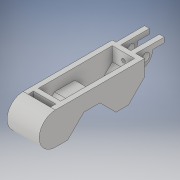
# Autodesk Inventor part: index
Saved by Autodesk Inventor 2019 (Build 230136000, 136)
## iProperties
Created: 2018-10-13
Part Number: index
Material: Generic
Document SubType Name: Modeling
Designer: jerem
Density: 1 g/cm^3
Appearance: Default
Author: jerem
Autodesk Inventor part; units mm, degrees
ref_plane "YZ Plane" through (0, 0, 0) normal (1, 0, 0) x (0, 1, 0)
ref_plane "XZ Plane" through (0, 0, 0) normal (0, 1, 0) x (-1, 0, 0)
sketch "Sketch2" plane through (0, 0, 0) normal (1, 0, 0) x (0, 1, 0)
  line L0 (0, 0) -> (0, -5)
  line L1 (13, 0) -> (13, -18)
  arc A0 (13, 0) -> (0, 0) centre (6.5, 0) ccw
  line L2 (-3.1385, 0) -> (18.8309, 0) projected
  line L3 (0, -54.8723) -> (0, 16.7287) projected
  line L4 (0, -5) -> (6.5, -11.5)
  line L5 (0, -5) -> (9.1924, -5) construction
  line L6 (6.5, -11.5) -> (6.5, -18)
  line L7 (6.5, -18) -> (0, -24.5)
  line L8 (6.5, -18) -> (15.6924, -18) construction
  line L9 (0, -24.5) -> (0, -29.5)
  line L10 (0, -29.5) -> (6.5, -36)
  line L11 (0, -29.5) -> (9.1924, -29.5) construction
  line L12 (13, -18) -> (13, -36)
  line L13 (13, -36) -> (13, -42.5)
  arc A1 (6.5, -36) -> (13, -42.5) centre (11.1419, -37.8581) ccw
  circle A2 centre (9.75, -40) radius 1.625
  dimension "d3" = 18
  dimension "d4" = 13
  dimension "d9" = 45
  dimension "d10" = 6.5
  dimension "d11" = 5
  dimension "d12" = 6.5
  dimension "d13" = 135
  dimension "d14" = 6.5
  dimension "d15" = 5
  dimension "d16" = 45
  dimension "d17" = 6.5
  dimension "d18" = 18
  dimension "d19" = 6.5
  dimension "d20" = 5
  dimension "d21" = 3.25
  dimension "d22" = 3.25
  dimension "d23" = 2.5
  constraints: 24 end point, 5 vertical, 4 point on circle, 3 centre point, 3 equal length, 3 horizontal, 2 point on line, 2 tangent, 1 collinear
  measures "d3" distance of L1.start L1.end
  measures "d4" distance between parallel lines of L1 L0
  measures "d9" angle of L4 L5
  measures "d10" horizontal distance of L4.end L0.end
  measures "d11" distance of L0.start L0.end
  measures "d12" distance of L4.end L6.end
  measures "d13" angle of L7 L8
  measures "d14" horizontal distance of L7.end L6.end
  measures "d15" distance of L7.end L9.end
  measures "d16" angle of L10 L11
  measures "d17" horizontal distance of L10.end L9.end
  measures "d18" distance of L1.end L12.end
  measures "d19" distance of L12.end L13.end
  measures "d20" radius of A1
  measures "d21" diameter of A2
  measures "d22" horizontal distance of A2.centre L13.end
  measures "d23" vertical distance of L13.end A2.centre
extrude "Extrusion1" add sketch "Sketch2" along normal mid plane 13 contours L2 L1 L12 L13 A1 L10 L3 L7 L6 L4 L0 | A0 L2
sketch "Sketch3" plane through (-6.5, 13, 0) normal (0, 1, 0) x (1, 0, 0)
  line L0 (0, 36) -> (13, 36) projected
  line L1 (0, 43) -> (1.5, 43)
  line L2 (1.5, 43) -> (1.5, 36)
  line L3 (1.5, 36) -> (0, 36)
  line L4 (0, 36) -> (0, 43)
  line L5 (0, 0) -> (0, 42.5) projected
  line L6 (3.5, 43) -> (7.5, 43)
  line L7 (7.5, 43) -> (7.5, 36)
  line L8 (7.5, 36) -> (3.5, 36)
  line L9 (3.5, 36) -> (3.5, 43)
  line L10 (9.5, 43) -> (13, 43)
  line L11 (13, 43) -> (13, 36)
  line L12 (13, 36) -> (9.5, 36)
  line L13 (9.5, 36) -> (9.5, 43)
  line L14 (13, 42.5) -> (13, 0) projected
  point P0 (6.5, 0)
  dimension "d47" = 1.5
  dimension "d48" = 7
  dimension "d49" = 4
  dimension "d50" = 7
  dimension "d51" = 2
  dimension "d52" = 7
  dimension "d53" = 2
  constraints: 24 end point, 6 parallel, 5 collinear, 3 horizontal, 3 perpendicular
  measures "d47" distance of L2.end L3.end
  measures "d48" distance of L1.end L2.end
  measures "d49" distance of L7.end L8.end
  measures "d50" distance of L6.end L7.end
  measures "d51" distance between parallel lines of L2 L9
  measures "d52" distance of L10.end L11.end
  measures "d53" distance between parallel lines of L13 L7
extrude "Extrusion2" cut sketch "Sketch3" against normal blind 13
ref_plane "Work Plane1" through (4.5, 0, 0) normal (1, 0, 0) x (0, 0, -1)
sketch "Sketch4" plane through (4.5, 0, 0) normal (1, 0, 0) x (0, 0, -1)
  arc A0 (0, 13) -> (0, 0) centre (0, 6.5) ccw projected
  line L0 (0, 13) -> (36, 13) projected
  line L1 (36, 13) -> (36, 6.5) projected
  line L2 (36, 6.5) -> (29.5, 0) projected
  line L3 (29.5, 0) -> (24.5, 0) projected
  line L4 (24.5, 0) -> (18, 6.5) projected
  line L5 (36, 13) -> (36, 6.5) projected
  line L6 (36, 6.5) -> (29.5, 0) projected
  line L7 (29.5, 0) -> (24.5, 0) projected
  line L8 (24.5, 0) -> (18, 6.5) projected
  line L9 (18, 6.5) -> (11.5, 6.5) projected
  line L10 (11.5, 6.5) -> (5, 0) projected
  line L11 (5, 0) -> (0, 0) projected
  arc A1 (0, 13) -> (0, 0) centre (0, 6.5) ccw projected
  line L12 (0, 13) -> (36, 13) projected
  line L13 (0, 13) -> (0, 2)
  line L14 (0, 2) -> (2.1716, 2)
  line L15 (4.1716, 2) -> (10.6716, 8.5)
  line L16 (4.1716, 2) -> (13.364, 2) construction
  line L17 (34, 13) -> (34, 7.3284)
  line L18 (34, 7.3284) -> (28.6716, 2)
  line L19 (34, 7.3284) -> (41.5355, 7.3284) construction
  line L20 (28.6716, 2) -> (25.3284, 2)
  line L21 (25.3284, 2) -> (18.8284, 8.5)
  line L22 (25.3284, 2) -> (34.5208, 2) construction
  line L23 (18.8284, 8.5) -> (10.6716, 8.5)
  line L24 (4.1716, 2) -> (4.1716, 13)
  line L25 (2.1716, 2) -> (2.1716, 13)
  line L26 (0, 13) -> (2.1716, 13)
  line L27 (4.1716, 13) -> (34, 13)
  dimension "d57" = 11
  dimension "d58" = 2
  dimension "d59" = 45
  dimension "d60" = 2
  dimension "d62" = 2
  dimension "d63" = 2
  dimension "d64" = 135
  dimension "d65" = 2
  dimension "d66" = 2
  dimension "d67" = 135
  dimension "d94" = 2
  dimension "d95" = 2
  constraints: 30 end point, 6 horizontal, 3 equal length, 3 perpendicular, 2 collinear, 1 point on line, 1 vertical
  measures "d57" distance of L12.start L13.end
  measures "d58" distance from line of L10 L15.start
  measures "d59" angle of L16 L15
  measures "d60" vertical distance of L9.end L15.end
  measures "d62" distance between parallel lines of L1 L17
  measures "d63" distance from line of L2 L17.end
  measures "d64" angle of L18 L19
  measures "d65" distance from line of L3 L18.end
  measures "d66" distance from line of L4 L20.end
  measures "d67" angle of L22 L21
  measures "d94" distance from line of L11 L15.start
  measures "d95" distance between parallel lines of L25 L24
extrude "Extrusion3" cut sketch "Sketch4" against normal blind 9 contours L0 L25 L14 L13 | L0 L17 L18 L20 L21 L23 L15 L24
sketch "Sketch5" plane through (4.5, 2, -4.1716) normal (0, 0, -1) x (-1, 0, 0)
  line L0 (0, 11) -> (0, 0) projected
  line L1 (9, 0) -> (9, 11) projected
  line L2 (0, 11) -> (0, 0) projected
  line L3 (0, 0) -> (9, 0) projected
  line L4 (9, 0) -> (9, 11) projected
  line L5 (0, 11) -> (9, 11) projected
  circle A0 centre (4.5, 8) radius 0.75
  circle A1 centre (4.5, 3) radius 0.75
  point P0 (4.5, -2)
  dimension "d72" = 1.5
  dimension "d73" = 4.5
  dimension "d74" = 3
  dimension "d75" = 1.5
  dimension "d76" = 3
  dimension "d77" = 4.5
  constraints: 2 centre point
  measures "d72" diameter of A0
  measures "d73" distance from line of L1 A0.centre
  measures "d74" distance from line of L5 A0.centre
  measures "d75" diameter of A1
  measures "d76" distance from line of L3 A1.centre
  measures "d77" distance from line of L1 A1.centre
extrude "Extrusion4" cut sketch "Sketch5" against normal blind 2 contours A0 | A1
sketch "Sketch6" plane through (1, 13, -36) normal (0, 0, -1) x (-1, 0, 0)
  line L0 (1, -15.6) -> (1, 2.6) projected
  line L1 (10.1, -13) -> (-8.1, -13) projected
  circle A0 centre (1, -3) radius 0.75
  line L2 (0, 0) -> (4, 0) projected
  circle A1 centre (1, -10) radius 0.75
  point P0 (1, -13)
  dimension "d80" = 1.5
  dimension "d81" = 3
  dimension "d82" = 1.5
  dimension "d83" = 3
  constraints: 2 centre point, 2 point on line
  measures "d80" diameter of A0
  measures "d81" distance from line of L2 A0.centre
  measures "d82" diameter of A1
  measures "d83" distance from line of L1 A1.centre
extrude "Extrusion5" cut sketch "Sketch6" against normal blind 9
sketch "Sketch7" plane through (3, 13, -36) normal (1, 0, 0) x (0, 0, -1)
  line L0 (6.5, 0) -> (0, 0) projected
  line L1 (6.5, 0) -> (11.5, 0)
  line L2 (11.5, 0) -> (11.5, -2)
  line L3 (11.5, -2) -> (6.5, -2)
  line L4 (6.5, -2) -> (6.5, 0)
  point P0 (-36, -13)
  dimension "d86" = 5
  dimension "d87" = 2
  constraints: 8 end point, 2 parallel, 1 collinear, 1 horizontal, 1 perpendicular
  measures "d86" distance of L2.end L3.end
  measures "d87" distance of L1.end L2.end
extrude "Extrusion6" add sketch "Sketch7" against normal blind 2
sketch "Sketch8" plane through (-5, 13, -42.5) normal (-1, 0, 0) x (0, 0, 1)
  line L0 (0, 0) -> (6.5, 0) projected
  line L1 (-5, -2) -> (0, -2)
  line L2 (0, -2) -> (0, 0)
  line L3 (0, 0) -> (-5, 0)
  line L4 (-5, 0) -> (-5, -2)
  point P0 (42.5, -13)
  dimension "d90" = 5
  dimension "d91" = 2
  constraints: 8 end point, 2 parallel, 1 horizontal, 1 perpendicular
  measures "d90" distance of L0.start L3.end
  measures "d91" distance of L0.start L1.end
extrude "Extrusion7" add sketch "Sketch8" against normal blind 2
body "Solid1"
